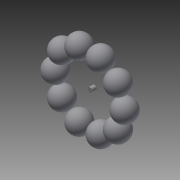
# Autodesk Inventor part: BallBearing
Saved by Autodesk Inventor 2015 (Build 190159000, 159)
## iProperties
Created: 2017-01-13
Part Number: BallBearing
Material: Generic
Document SubType Name: Modeling
Designer: 1esh9
Density: 1 g/cm^3
Appearance: Default
Author: 1esh9
Autodesk Inventor part; units mm, degrees
ref_plane "YZ Plane" through (0, 0, 0) normal (1, 0, 0) x (0, 1, 0)
ref_plane "XZ Plane" through (0, 0, 0) normal (0, 1, 0) x (-1, 0, 0)
ref_plane "XY Plane" through (0, 0, 0) normal (0, 0, 1) x (1, 0, 0)
sketch "Sketch3" plane through (0, 0, 0) normal (0, 0, 1) x (1, 0, 0)
  line L0 (0, 4.385) -> (0, -4.7892)
  line L1 (0, 0) -> (7.68, 0)
  line L2 (7.68, 2.375) -> (7.68, -2.375)
  arc A0 (7.68, -2.375) -> (7.68, 2.375) centre (7.68, 0) ccw
  dimension "d6" = 7.68
  dimension "d7" = 4.75
  constraints: 6 end point, 2 point on circle, 2 vertical, 1 centre point, 1 coincident, 1 horizontal, 1 midpoint
  measures "d6" distance of L1.start L1.end
  measures "d7" diameter of A0
revolve "Revolution2" add sketch "Sketch3" angle 360 about axis through (7.68, 2.375, 0) along (0, -1, 0)
pattern_circular "Circular Pattern1" count 10 over 360 about axis through (0, -10, 0) along (0, 1, 0) of "Revolution2"
sketch "Sketch4" plane through (0, 0, 0) normal (0, 1, 0) x (-1, 0, 0)
  circle A0 centre (0, 0) radius 0.5
  dimension "d12" = 1
  constraints: 1 centre point, 1 coincident
  measures "d12" diameter of A0
extrude "Extrusion1" add sketch "Sketch4" along normal blind 1
body "Solid2"
